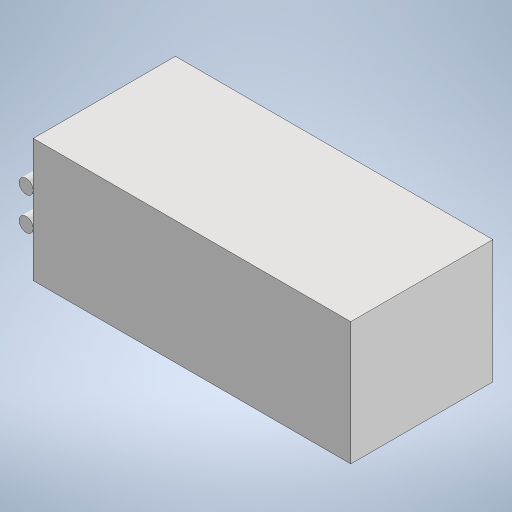
# Autodesk Inventor part: Temp - Battery
Saved by Autodesk Inventor 2023.2 (Build 272271000, 271)
## iProperties
Created: 2023-06-09
Part Number: Temp - Battery
Material: Generic
Document SubType Name: Modeling
Designer: Nathan Cai
Mass: 106 g
Surface Area: 96.5776 cm^2
Volume: 52.6841 cm^3
Density: 2.01199 g/cm^3
Appearance: Default
Author: Nathan Cai
Autodesk Inventor part; units mm, degrees
ref_plane "YZ Plane" through (0, 0, 0) normal (1, 0, 0) x (0, 1, 0)
ref_plane "XZ Plane" through (0, 0, 0) normal (0, 1, 0) x (-1, 0, 0)
ref_plane "XY Plane" through (0, 0, 0) normal (0, 0, 1) x (1, 0, 0)
sketch "Sketch1" plane through (0, 0, 0) normal (0, 1, 0) x (-1, 0, 0)
  line L0 (0, 0) -> (67, 0)
  line L1 (67, 0) -> (67, -30)
  line L2 (67, -30) -> (0, -30)
  line L3 (0, -30) -> (0, 0)
  dimension "d0" = 67
  dimension "d1" = 30
  constraints: 8 end point, 2 parallel, 1 horizontal, 1 perpendicular
  measures "d0" distance of L1.end L2.end
  measures "d1" distance between parallel lines of L0 L2
extrude "Extrusion1" add sketch "Sketch1" along normal blind 26
sketch "Sketch2" plane through (-67, 0, 0) normal (0, 0, 1) x (1, 0, 0)
  circle A0 centre (-1.5, 16.475) radius 1.5
  line L0 (0, 0) -> (0, 26) projected
  line L1 (0, 26) -> (67, 26) projected
  line L2 (0, 0) -> (0, 26) projected
  line L3 (0, 13) -> (5.0993, 13) construction
  circle A1 centre (-1.5, 9.525) radius 1.5
  point P0 (67, 0)
  dimension "d4" = 3
  dimension "d5" = 9.525
  constraints: 2 centre point, 2 end point, 1 horizontal, 1 midpoint, 1 symmetric about line, 1 tangent, 1 other
  measures "d4" diameter of A0
  measures "d5" distance from line of L1 A0.centre
extrude "Extrusion2" add sketch "Sketch2" against normal up to surface (30 mm away)
body "Solid1"
